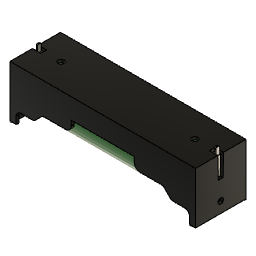
18650 Battery and Holder 02 v2 (Autodesk Fusion 360 design; units mm, degrees)
Autodesk Fusion 360 part; units mm, degrees
note: some values were not read from the file. Set by a fixed rule: which face or edge a step refers to.
sketch "Sketch1" plane through (0, 0, 0) normal (0, 0, 1) x (1, 0, 0) in component "Battery Assembly"
  line L0 (-0.0012, -0.0018) -> (77.2488, -0.0018)
  line L1 (77.2488, -0.0018) -> (77.2488, -21.0018)
  line L2 (77.2488, -21.0018) -> (-0.0012, -21.0018)
  line L3 (-0.0012, -21.0018) -> (-0.0012, -0.0018)
  dimension "d325_1" = 77.25
  dimension "d326_1" = 21
  constraint horizontal L0
  constraint vertical L1
  constraint horizontal L2
  constraint vertical L3
  measures "d325_1" distance of L0.start L0.end
  measures "d326_1" distance of L0.start L2.end
extrude "Extrude1" add sketch "Sketch1" against normal blind 22 makes body 1 in component "Battery Assembly"
shell "Shell1" thickness 1.2 removed faces 1 at (25.7488, -14.0018, -22) on bodies 1 in component "Battery Assembly"
sketch "Sketch3" plane through (0, -21.0018, 0) normal (0, -1, 0) x (1, 0, 0) in component "Battery Assembly"
  line L0 (77.2488, 0) -> (-0.0012, 0)
  line L1 (-0.0012, 0) -> (-0.0012, -22)
  line L2 (-0.0012, -22) -> (77.2488, -22)
  line L3 (77.2488, -22) -> (77.2488, 0)
  line L4 (77.2488, -22) -> (74.7488, -22)
  line L5 (74.7488, -22) -> (74.7488, -16.5)
  line L6 (74.7488, -16.5) -> (67.2488, -16.5)
  line L7 (67.2488, -16.5) -> (63.7132, -12.9645)
  line L8 (63.7132, -12.9645) -> (51.7132, -12.9645)
  line L9 (51.7132, -12.9645) -> (51.7132, -8.4645)
  line L10 (51.7132, -8.4645) -> (25.5332, -8.4645)
  line L11 (25.5332, -8.4645) -> (25.5332, -12.9645)
  line L12 (25.5332, -12.9645) -> (13.5332, -12.9645)
  line L13 (13.5332, -12.9645) -> (9.9977, -16.5)
  line L14 (9.9977, -16.5) -> (2.4977, -16.5)
  line L15 (2.4977, -16.5) -> (2.4977, -22)
  line L16 (2.4977, -22) -> (-0.0012, -22)
  dimension "d444" = 2.5
  dimension "d445" = 5.5
  dimension "d446" = 7.5
  dimension "d447" = 5
  dimension "d448" = 12
  dimension "d449" = 135
  dimension "d450" = 135
  dimension "d451" = 4.5
  dimension "d452" = 26.18
  dimension "d453" = 135
  constraint coincident L3 L2.end
  constraint perpendicular L3 L4
  constraint collinear L2 L4
  constraint perpendicular L4 L5
  constraint perpendicular L5 L6
  constraint perpendicular L8 L9
  constraint perpendicular L9 L10
  constraint perpendicular L10 L11
  constraint equal L9 L11
  constraint perpendicular L11 L12
  constraint equal L8 L12
  constraint equal L7 L13
  constraint horizontal L14
  constraint equal L6 L14
  constraint perpendicular L14 L15
  constraint equal L5 L15
  constraint coincident L1.end L2.start
  measures "d444" distance of L2.end L4.end
  measures "d445" distance of L4.end L5.end
  measures "d446" distance of L5.end L6.end
  measures "d447" distance of L6.end L7.end
  measures "d448" distance of L7.end L8.end
  measures "d449" angle of L6 L7
  measures "d450" angle of L7 L8
  measures "d451" distance of L8.end L9.end
  measures "d452" distance of L9.end L10.end
  measures "d453" angle of L13 L14
extrude "Extrude10" cut sketch "Sketch3" against normal up to surface (21 mm away) contours L2 L5 L6 L7 L8 L9 L10 L11 L12 L13 L14 L15 bodies 1 in component "Battery Assembly"
fillet "Fillet3" radius 2 4 edges at (74.7488, -20.4018, -16.5) (2.4977, -20.4018, -16.5) (2.4977, -0.6018, -16.5) (74.7488, -0.6018, -16.5) on bodies 1 in component "Battery Assembly"
fillet "Fillet3" radius 1.5 4 edges at (67.2488, -20.4018, -16.5) (67.2488, -0.6018, -16.5) (9.9977, -20.4018, -16.5) (9.9977, -0.6018, -16.5) on bodies 1 in component "Battery Assembly"
fillet "Fillet3" radius 1.25 4 edges at (63.7132, -20.4018, -12.9645) (63.7132, -0.6018, -12.9645) (13.5332, -20.4018, -12.9645) (13.5332, -0.6018, -12.9645) on bodies 1 in component "Battery Assembly"
fillet "Fillet3" radius 2.5 4 edges at (25.5332, -20.4018, -12.9645) (25.5332, -0.6018, -12.9645) (51.7132, -20.4018, -12.9645) (51.7132, -0.6018, -12.9645) on bodies 1 in component "Battery Assembly"
fillet "Fillet5" radius 5 2 edges at (38.6238, -19.8018, -1.2) (38.6238, -1.2018, -1.2) on bodies 1 in component "Battery Assembly"
sketch "Sketch4" plane through (77.2488, 0, 0) normal (1, 0, 0) x (0, 1, 0) in component "Battery Assembly"
  line L0 (-0.0018, 0) -> (-21.0018, 0)
  line L1 (-21.0018, 0) -> (-21.0018, -22)
  line L2 (-21.0018, -22) -> (-0.0018, -22)
  line L3 (-0.0018, -22) -> (-0.0018, 0)
  circle A0 centre (-10.5018, -17) radius 1.125
  line L4 (-10.5018, -22) -> (-10.5018, 0) construction
  line L5 (-10.5018, -22) -> (-10.5018, -17) construction
  line L6 (-10.5018, 0) -> (-10.5018, -9) construction
  line L7 (-10.5018, -9) -> (-11.5018, -9)
  line L8 (-11.5018, -9) -> (-11.7018, 0)
  line L9 (-10.5018, 0) -> (-11.7018, 0)
  line L10 (-9.5018, -9) -> (-9.3018, 0)
  line L11 (-10.5018, -9) -> (-9.5018, -9)
  line L12 (-10.5018, 0) -> (-9.3018, 0)
  dimension "d460" = 2.25
  dimension "d461" = 5
  dimension "d462" = 9
  dimension "d463" = 1.2
  dimension "d464" = 1
  constraint midpoint L2 L4.start
  constraint midpoint L0 L4.end
  constraint coincident L4 A0.centre
  constraint coincident A0.centre L4
  constraint coincident L4 L6.end
  constraint perpendicular L6 L7
  constraint coincident L0 L8.end
  constraint symmetric L6.start L4 L9.start
  constraint symmetric L4 L6.end L7.start
  constraint symmetric L4 L7.end L10.start
  constraint symmetric L4 L8.end L10.end
  constraint coincident A0.centre L5.end
  measures "d460" diameter of A0
  measures "d461" distance of L4.start A0.centre
  measures "d462" distance of L4.end L6.end
  measures "d463" distance of L4.end L8.end
  measures "d464" distance of L6.end L7.end
extrude "Extrude11" cut sketch "Sketch4" against normal up to surface (77.25 mm away) contours A0 bodies 1 in component "Battery Assembly"
extrude "Extrude12" cut sketch "Sketch4" against normal blind 3.5 contours L0 L7 L8 L9 L10 L11 L12 bodies 1 in component "Battery Assembly"
sketch "Sketch5" plane through (-0.0012, 0, 0) normal (-1, 0, 0) x (0, -1, 0) in component "Battery Assembly"
  circle A0 centre (10.5018, -17) radius 1.125
  line L0 (21.0018, 0) -> (0.0018, 0)
  line L1 (0.0018, 0) -> (0.0018, -22)
  line L2 (0.0018, -22) -> (21.0018, -22)
  line L3 (21.0018, -22) -> (21.0018, 0)
  line L4 (10.5018, -22) -> (10.5018, 0) construction
  line L5 (11.5018, -9) -> (9.5018, -9) construction
  line L6 (10.5018, -9) -> (10.5018, 0) construction
  line L7 (10.5018, -9) -> (11.5018, -9)
  line L8 (11.5018, -9) -> (11.7018, 0)
  line L9 (11.7018, 0) -> (10.5018, 0)
  line L10 (9.5018, -9) -> (9.3018, 0)
  line L11 (10.5018, -9) -> (9.5018, -9)
  line L12 (9.3018, 0) -> (10.5018, 0)
  dimension "d470" = 9
  dimension "d471" = 1.2
  dimension "d472" = 1
  constraint midpoint L2 L4.start
  constraint midpoint L0 L4.end
  constraint midpoint L5 L6.start
  constraint coincident L4 L6.end
  constraint perpendicular L0 L6
  constraint coincident L5.start L7.end
  constraint coincident L0 L8.end
  constraint perpendicular L4 L9
  constraint symmetric L7.start L6 L11.start
  constraint symmetric L4.end L6 L9.end
  constraint symmetric L6 L5.start L5.end
  constraint symmetric L6 L8.end L10.end
  measures "d470" distance of L6.start L4.end
  measures "d471" distance of L4.end L8.end
  measures "d472" distance of L6.start L5.start
extrude "Extrude13" cut sketch "Sketch5" against normal blind 3.5 contours L0 L7 L8 L9 L10 L11 L12 bodies 1 in component "Battery Assembly"
sketch "Sketch2" plane through (77.2488, 0, 0) normal (1, 0, 0) x (0, 1, 0) in component "Battery Assembly"
  line L0 (-11.7018, 0) -> (-21.0018, 0)
  line L1 (-21.0018, 0) -> (-21.0018, -22)
  line L2 (-21.0018, -22) -> (-0.0018, -22)
  line L3 (-0.0018, -22) -> (-0.0018, 0)
  line L4 (-10.5018, 0) -> (-10.5018, -22) construction
  line L5 (-19.8018, -6.2) -> (-19.8018, -22) construction
  circle A0 centre (-10.5018, -11) radius 9
  line L6 (-11.5018, -9) -> (-11.7018, 0)
  line L7 (-0.0018, 0) -> (-9.3018, 0)
  line L8 (-9.3018, 0) -> (-9.5018, -9)
  line L9 (-9.5018, -9) -> (-11.5018, -9)
  circle A1 centre (-10.5018, -17) radius 1.125
  line L10 (-11.7018, 0) -> (-9.3018, 0)
  line L11 (-21.0018, -11) -> (-6, -11) construction
  line L12 (-11.6752, -1.2) -> (-14.8018, -1.2)
  line L13 (-6.2018, -1.2) -> (-9.3285, -1.2)
  dimension "d331_1" = 18
  constraint midpoint L2 L4.end
  constraint midpoint L4 A0.centre
  constraint midpoint L4.start L10
  constraint midpoint L1 L11.start
  constraint perpendicular L4 L11
  measures "d331_1" diameter of A0
extrude "Extrude2" add sketch "Sketch2" against normal blind 65 from surface at -6 separate body contours A0 L6 L8 L9 | A0 L6 L8 L9 | A1 makes body 2 in component "Battery Assembly"
sketch "Sketch3 (2)" plane through (0, 0, -1.2) normal (0, 0, -1) x (1, 0, 0) in component "Battery Assembly"
  line L0 (76.0621, 19.821) -> (1.2121, 19.821)
  line L1 (1.2121, 19.821) -> (1.2121, 1.221)
  line L2 (1.2121, 1.221) -> (76.0621, 1.221)
  line L3 (76.0621, 1.221) -> (76.0621, 19.821)
  line L4 (1.2121, 13.771) -> (5.9621, 13.771)
  line L5 (5.9621, 13.771) -> (5.9621, 7.271)
  line L6 (5.9621, 7.271) -> (1.2121, 7.271)
  line L7 (1.2121, 7.271) -> (1.2121, 13.771)
  line L8 (76.0621, 14.071) -> (71.3121, 14.071)
  line L9 (71.3121, 14.071) -> (71.3121, 7.571)
  line L10 (71.3121, 7.571) -> (76.0621, 7.571)
  line L11 (76.0621, 7.571) -> (76.0621, 14.071)
  line L12 (3.5871, 13.771) -> (3.5871, 19.521) construction
  line L13 (73.6871, 14.071) -> (73.6871, 19.821) construction
  line L14 (1.1988, 9.3285) -> (1.1988, 6.2018)
  line L15 (76.0488, 6.2018) -> (76.0488, 9.3285)
  line L16 (1.1481, 10.521) -> (76.0621, 10.521) construction
  circle A0 centre (10.7488, 10.521) radius 1.25
  line L17 (-0.0012, 21.0018) -> (-0.0012, 0.0018) construction
  line L18 (10.7488, 10.521) -> (-0.0012, 10.5018) construction
  circle A1 centre (66.4988, 10.521) radius 1.25
  line L19 (77.2488, 0.0018) -> (77.2488, 21.0018) construction
  line L20 (66.4988, 10.521) -> (77.2488, 10.5018) construction
  line L21 (1.1988, 11.6752) -> (3.4988, 11.6752)
  line L22 (3.4988, 11.6752) -> (3.4988, 9.3285)
  line L23 (3.4988, 9.3285) -> (1.1988, 9.3285)
  line L24 (76.0488, 9.3285) -> (73.7488, 9.3285)
  line L25 (73.7488, 9.3285) -> (73.7488, 11.6752)
  line L26 (73.7488, 11.6752) -> (76.0488, 11.6752)
  line L27 (76.0488, 11.6752) -> (76.0488, 14.8018)
  line L28 (1.1988, 6.2018) -> (76.0488, 6.2018)
  line L29 (76.0488, 14.8018) -> (1.1988, 14.8018)
  line L30 (1.1988, 14.8018) -> (1.1988, 11.6752)
  dimension "d327_1" = 6.5
  dimension "d328_1" = 6.5
  dimension "d332_1" = 5.75
  dimension "d333_1" = 4.75
  dimension "d144" = 2.5
  dimension "d145" = 10.75
  dimension "d146" = 2.5
  dimension "d147" = 10.75
  constraint horizontal L4
  constraint vertical L5
  constraint horizontal L6
  constraint vertical L7
  constraint coincident L1 L4.start
  constraint horizontal L8
  constraint vertical L9
  constraint horizontal L10
  constraint vertical L11
  constraint coincident L3 L8.start
  constraint midpoint L4 L12.start
  constraint perpendicular L0 L12
  constraint equal L4 L8
  constraint midpoint L8 L13.start
  constraint coincident L0 L13.end
  constraint perpendicular L0 L13
  constraint equal L12 L13
  constraint midpoint L3 L16.end
  constraint coincident L16 A0.centre
  constraint coincident A0.centre L18.start
  constraint midpoint L17 L18.end
  constraint coincident L16 A1.centre
  constraint coincident A1.centre L20.start
  constraint midpoint L19 L20.end
  constraint horizontal L16
  measures "d327_1" distance of L4.start L6.end
  measures "d328_1" distance of L8.start L10.end
  measures "d332_1" distance of L12.start L12.end
  measures "d333_1" distance of L5.end L6.end
  measures "d144" diameter of A0
  measures "d145" horizontal distance of A0.centre L18.end
  measures "d146" diameter of A1
  measures "d147" horizontal distance of A1.centre L20.end
extrude "Extrude3" add sketch "Sketch3 (2)" along normal blind 16 separate body contours L3 L8 L10 L11 L15 L24 L25 L26 L27 | L8 L9 L10 L15 L24 L25 L26 L27 | L1 L4 L5 L6 L7 L21 L22 L23 | L1 L7 L21 L22 L23 makes body 3 at (76.0621, -9.7377, -6.5333) makes body 4 at (5.9621, -11.6044, -6.5333) in component "Battery Assembly"
sketch "Sketch6" plane through (0, 0, -1.2) normal (0, 0, 1) x (-1, 0, 0) in component "Battery Assembly"
  line L0 (-76.0621, 14.071) -> (-76.0621, 7.571)
  line L1 (-76.0621, 7.571) -> (-71.3121, 7.571)
  line L2 (-71.3121, 7.571) -> (-71.3121, 14.071)
  line L3 (-71.3121, 14.071) -> (-76.0621, 14.071)
  line L4 (-76.0457, 11.25) -> (-75.5457, 11.25)
  line L5 (-75.5457, 11.25) -> (-75.5457, 9.75)
  line L6 (-75.5457, 9.75) -> (-76.0457, 9.75)
  line L7 (-76.0457, 9.75) -> (-76.0457, 11.25)
  line L8 (-1.7148, 11.25) -> (-1.2148, 11.25)
  line L9 (-1.2148, 11.25) -> (-1.2148, 9.75)
  line L10 (-1.2148, 9.75) -> (-1.7148, 9.75)
  line L11 (-1.7148, 9.75) -> (-1.7148, 11.25)
  dimension "d477" = 0.5
  dimension "d478" = 1.5
  dimension "d479" = 1.5
  dimension "d480" = 0.5
  constraint horizontal L4
  constraint vertical L5
  constraint horizontal L6
  constraint vertical L7
  constraint horizontal L8
  constraint vertical L9
  constraint horizontal L10
  constraint vertical L11
  measures "d477" distance of L8.start L8.end
  measures "d478" distance of L8.start L10.end
  measures "d479" distance of L4.start L6.end
  measures "d480" distance of L4.start L4.end
extrude "Extrude14" add sketch "Sketch6" along normal blind 3.25 contours L4 L5 L6 L7 | L8 L9 L10 L11 bodies 3 4 in component "Battery Assembly"
fillet "Fillet4" radius 0.5 4 edges at (75.7957, -9.75, 2.05) (75.7957, -11.25, 2.05) (1.4648, -9.75, 2.05) (1.4648, -11.25, 2.05) on bodies 3 4 in component "Battery Assembly"
extrude "Extrude4" cut sketch "Sketch3 (2)" against normal up to surface (1.2 mm away) contours A0 | A1 bodies 1 in component "Battery Assembly"
chamfer "Chamfer1" distance 2.5 angle 45 2 edges at (71.3121, -10.821, -17.2) (5.9621, -10.521, -17.2) on bodies 3 4 in component "Battery Assembly"
fillet "Fillet2" radius 0.5 2 faces at (76.8488, -13.6018, -22) (0.3988, -7.4018, -22) on bodies 1 in component "Battery Assembly"
fillet "Fillet1" radius 1 2 edges at (6.2488, -18.8928, -7.7455) (71.2488, -18.8928, -14.2545) on bodies 2 in component "Battery Assembly"
sketch "Sketch4 (2)" plane through (71.2488, 0, 0) normal (1, 0, 0) x (0, 1, 0) in component "Battery Assembly"
  circle A0 centre (-10.5018, -11) radius 8
  circle A1 centre (-10.5018, -11) radius 7.875
  dimension "d428" = 15.75
  constraint concentric A0 A1
  measures "d428" diameter of A1
extrude "Extrude5" cut sketch "Sketch4 (2)" against normal blind 0.2 contours A1 bodies 2 in component "Battery Assembly"
extrude "Extrude6" add sketch "Sketch4 (2)" along normal blind 0.1 separate body contours A1 makes body 5 in component "Battery Assembly"
sketch "Sketch5 (2)" plane through (6.2488, 0, 0) normal (-1, 0, 0) x (0, -1, 0) in component "Battery Assembly"
  circle A0 centre (10.5018, -11) radius 8
  circle A1 centre (10.5018, -11) radius 6
  circle A2 centre (10.5018, -11) radius 4
  dimension "d433" = 12
  dimension "d434" = 8
  constraint concentric A0 A1
  constraint concentric A1 A2
  measures "d433" diameter of A1
  measures "d434" diameter of A2
extrude "Extrude7" cut sketch "Sketch5 (2)" against normal blind 0.6 contours A1 bodies 2 in component "Battery Assembly"
extrude "Extrude8" add sketch "Sketch5 (2)" along normal blind 0.1 separate body contours A1 makes body 6 in component "Battery Assembly"
extrude "Extrude9" add sketch "Sketch5 (2)" along normal blind 0.1 separate body contours A2 makes body 7 in component "Battery Assembly"
component "Battery Assembly" placed x (1, 0, 0) y (0, 1, 0) z (0, 0, 1) at (0, 0, 0)
equation "d332_1 = ( d326_1 - 3 mm - 6.5 mm ) / 2"
equation "Wall_Thickness = 2 mm"
equation "Pillar_Width = 8 mm"
equation "d146 = d144"
equation "d147 = d145"
equation "d223 = Wall_Thickness / 2"
equation "d463 = ( 2.4 / 2 ) * 1 mm"
equation "d464 = ( 2 / 2 ) * 1 mm"
equation "d471 = ( 2.4 / 2 ) * 1 mm"
named bodies: "Battery Holder", "18650 Battery", "Contact 1", "Contact 2", "Negative Terminal", "Insulation 1", "Positive Terminal"
